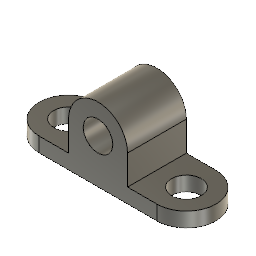
A4 HomeWork 2 (Autodesk Fusion 360 design; units mm, degrees)
Autodesk Fusion 360 part; units mm, degrees
sketch "Sketch1" plane through (0, 0, 0) normal (0, 1, 0) x (1, 0, 0)
  line L0 (0, 0) -> (80, 0)
  line L1 (80, 0) -> (80, -10)
  line L2 (80, -10) -> (0, -10)
  line L3 (0, -10) -> (0, 0)
  dimension "d1" = 10
  dimension "d2" = 80
  constraint horizontal L0
  constraint vertical L1
  constraint horizontal L2
  constraint vertical L3
  constraint coincident L0.start L3.end
  measures "d1" distance of L0 L2
  measures "d2" distance of L1 L3
  measures "d19" diameter of L0.start
extrude "Extrude1" add sketch "Sketch1" along normal blind 40
sketch "Sketch2" plane through (0, 0, 0) normal (0, -1, 0) x (1, 0, 0)
  line L0 (80, 10) -> (0, 10)
  line L1 (0, 10) -> (0, 0)
  line L2 (0, 0) -> (80, 0)
  line L3 (80, 0) -> (80, 10)
  line L4 (0, 10) -> (20, 10)
  line L5 (20, 10) -> (60, 10)
  line L6 (20, 10) -> (20, 30)
  line L7 (20, 30) -> (60, 30)
  line L8 (60, 30) -> (60, 10)
  circle A0 centre (40, 30) radius 20
  circle A1 centre (40, 30) radius 10
  dimension "d5" = 20
  dimension "d6" = 40
  dimension "d7" = 20
  dimension "d8" = 40
  dimension "d9" = 20
  constraint coincident L0.end L1.start
  constraint perpendicular L1 L4
  constraint parallel L0 L5
  constraint perpendicular L4 L6
  constraint perpendicular L6 L7
  constraint midpoint L7 A0.centre
  constraint concentric A0 A1
  measures "d5" distance of L0.end L4.end
  measures "d6" distance of L4.end L5.end
  measures "d7" distance of L4.end L6.end
  measures "d8" diameter of A0
  measures "d9" diameter of A1
extrude "Extrude2" add sketch "Sketch2" against normal blind 40 contours L0 L5 L8 A0 | L0 L5 L6 A0 | L7 A0 A1 | L7 A0 A1
sketch "Sketch3" plane through (0, 0, 10) normal (0, 0, 1) x (-1, 0, 0)
  line L0 (-60, -40) -> (-60, 0)
  line L1 (-60, 0) -> (-80, 0)
  line L2 (-80, 0) -> (-80, -40)
  line L3 (-80, -40) -> (-60, -40)
  circle A0 centre (-80, -20) radius 20
  circle A1 centre (-80, -20) radius 10
  dimension "d12" = 40
  dimension "d13" = 20
  constraint midpoint L2 A0.centre
  constraint concentric A0 A1
  measures "d12" diameter of A0
  measures "d13" diameter of A1
extrude "Extrude3" add sketch "Sketch3" against normal blind 10 contours L2 A0 A1 picked at (-90.5572, -7.1612)
hole "Hole1" at (80, 20, 10) direction (0, 0, -1) diameter 20 depth 20 tip angle 118
sketch "Sketch4" plane through (0, 0, 10) normal (0, 0, 1) x (-1, 0, 0)
  line L0 (-20, 0) -> (-20, -40)
  line L1 (-20, -40) -> (0, -40)
  line L2 (0, -40) -> (0, 0)
  line L3 (0, 0) -> (-20, 0)
  circle A0 centre (0, -20) radius 20
  circle A1 centre (0, -20) radius 10
  dimension "d19" = 40
  dimension "d20" = 20
  constraint midpoint L2 A0.centre
  constraint concentric A0 A1
  measures "d19" diameter of A0
  measures "d20" diameter of A1
extrude "Extrude4" add sketch "Sketch4" against normal blind 10 contours L2 A0 A1 picked at (16.5988, -20.9488)
hole "Hole2" at (0, 20, 10) direction (0, 0, -1) diameter 20 depth 100 tip angle 118
